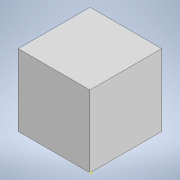
# Autodesk Inventor part: pawn-2
Saved by Autodesk Inventor 2021 (Build 250183000, 183)
## iProperties
Created: 2021-01-10
Part Number: pawn-2
Material: Generic
Document SubType Name: Modeling
Designer: Luke Kamols
Density: 1 g/cm^3
Appearance: Default
Author: Luke Kamols
Autodesk Inventor part; units mm, degrees
ref_plane "YZ Plane" through (0, 0, 0) normal (1, 0, 0) x (0, 1, 0)
ref_plane "XZ Plane" through (0, 0, 0) normal (0, 1, 0) x (-1, 0, 0)
ref_plane "XY Plane" through (0, 0, 0) normal (0, 0, 1) x (1, 0, 0)
sketch "Sketch1" plane through (0, 0, 0) normal (0, 1, 0) x (-1, 0, 0)
  point P0 (0, 0)
sketch "Sketch2" plane through (0, 0, 0) normal (0, 1, 0) x (-1, 0, 0)
  line L0 (0, 0) -> (16, 0)
  line L1 (16, 0) -> (16, -16)
  line L2 (16, -16) -> (0, -16)
  line L3 (0, -16) -> (0, 0)
  line L4 (0, 0) -> (0, -8)
  dimension "d1" = 16
  dimension "d2" = 16
  constraints: 10 end point, 2 parallel, 1 horizontal, 1 midpoint, 1 perpendicular
  measures "d1" distance of L1.end L2.end
  measures "d2" distance of L0.end L1.end
extrude "Extrusion1" add sketch "Sketch2" along normal blind 16
sketch "Sketch3" plane through (0, 0, 0) normal (0, -1, 0) x (1, 0, 0)
  line L0 (-16, 0) -> (0, 0) projected
  line L1 (-16, -16) -> (-16, 0) projected
  line L2 (0, 0) -> (0, -16) projected
  line L3 (-1.5, -8) -> (-1.5, -9.8)
  line L4 (-1.5, -9.8) -> (-14.5, -9.8)
  line L5 (-14.5, -9.8) -> (-14.5, -6.2)
  line L6 (-14.5, -6.2) -> (-1.5, -6.2)
  line L7 (-1.5, -6.2) -> (-1.5, -8)
  line L8 (-8, -1.5) -> (-6.2, -1.5)
  line L9 (-6.2, -1.5) -> (-6.2, -14.5)
  line L10 (-6.2, -14.5) -> (-9.8, -14.5)
  line L11 (-9.8, -14.5) -> (-9.8, -1.5)
  line L12 (-9.8, -1.5) -> (-8, -1.5)
  point P0 (-6.2, -6.2)
  point P1 (-9.8, -6.2)
  point P2 (-9.8, -9.8)
  point P3 (-6.2, -9.8)
  dimension "d22" = 13
  dimension "d23" = 3.6
  dimension "d25" = 1.8
  dimension "d26" = 13
  dimension "d27" = 3.6
  constraints: 20 end point, 7 perpendicular, 1 point on line
  measures "d22" distance of L3.end L4.end
  measures "d23" distance of L4.end L5.end
  measures "d25" distance of L8.start L8.end
  measures "d26" distance of L8.end L9.end
  measures "d27" distance of L9.end L10.end
extrude "Extrusion2" cut sketch "Sketch3" against normal blind 13
body "Solid1"
